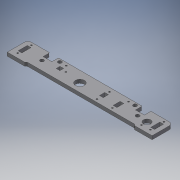
# Autodesk Inventor part: A8-0009
Saved by Autodesk Inventor 2016 SP2 (Build 200236200, 236)
## iProperties
Created: 2017-04-22
Part Number: A8-0009
Material: Generic
Document SubType Name: Modeling
Designer: EV
Density: 1 g/cm^3
Appearance: Default
Author: EV
Autodesk Inventor part; units mm, degrees
sketch "Sketch1" plane through (0, 0, 0) normal (0, 1, 0) x (-1, 0, 0)
  line L0 (-165, 47) -> (-165, 8)
  line L1 (165, 8) -> (165, 47)
  line L2 (-78, 0) -> (95.3, 0)
  line L3 (95.3, 0) -> (95.3, 15)
  line L4 (95.3, 15) -> (115.5, 15)
  line L5 (115.5, 15) -> (115.5, 0)
  line L6 (-115.5, 0) -> (-115.5, 15)
  line L7 (-115.5, 15) -> (-95.3, 15)
  line L8 (-95.3, 15) -> (-95.3, 0)
  line L9 (125, 47) -> (122, 44)
  line L10 (122, 44) -> (-122, 44)
  line L11 (-122, 44) -> (-125, 47)
  line L12 (0, 0) -> (0, 44) construction
  line L13 (165, 47) -> (125, 47)
  line L14 (-125, 47) -> (-165, 47)
  line L15 (115.5, 0) -> (157, 0)
  line L16 (-157, 0) -> (-115.5, 0)
  line L17 (-95.3, 0) -> (95.3, 0)
  line L18 (155.4, 11) -> (146.9, 11)
  line L19 (146.9, 11) -> (146.9, 32)
  line L20 (146.9, 32) -> (155.4, 32)
  line L21 (155.4, 32) -> (155.4, 11)
  line L22 (-146.9, 11) -> (-155.4, 11)
  line L23 (-155.4, 11) -> (-155.4, 32)
  line L24 (-155.4, 32) -> (-146.9, 32)
  line L25 (-146.9, 32) -> (-146.9, 11)
  line L26 (77, 15) -> (68.5, 15)
  line L27 (68.5, 15) -> (68.5, 23.5)
  line L28 (68.5, 23.5) -> (77, 23.5)
  line L29 (77, 23.5) -> (77, 15)
  line L30 (-25.6785, 15.5) -> (-34.1785, 15.5)
  line L31 (-34.1785, 15.5) -> (-34.1785, 27.5)
  line L32 (-34.1785, 27.5) -> (-25.6785, 27.5)
  line L33 (-25.6785, 27.5) -> (-25.6785, 15.5)
  line L34 (-60.7209, 15.5) -> (-69.2209, 15.5)
  line L35 (-69.2209, 15.5) -> (-69.2209, 31.5)
  line L36 (-69.2209, 31.5) -> (-60.7209, 31.5)
  line L37 (-60.7209, 31.5) -> (-60.7209, 15.5)
  arc A0 (157, 0) -> (165, 8) centre (157, 8) ccw
  arc A1 (-165, 8) -> (-157, 0) centre (-157, 8) ccw
  dimension "d0" = 330
  dimension "d1" = 47
  dimension "d2" = 45
  dimension "d3" = 3
  dimension "d4" = 40
  dimension "d5" = 49.5
  dimension "d6" = 20.2
  dimension "d8" = 15
  dimension "d9" = 11
  dimension "d10" = 9.6
  dimension "d11" = 8.5
  dimension "d12" = 21
  dimension "d13" = 8.5
  dimension "d14" = 8.5
  dimension "d15" = 8.5
  dimension "d16" = 12
  dimension "d17" = 8.5
  dimension "d18" = 16
  dimension "d19" = 95.7791
  dimension "d20" = 130.8215
  dimension "d21" = 88
  dimension "d22" = 15
  dimension "d23" = 15.5
  dimension "d24" = 15.5
  dimension "d25" = 8
  constraints: 76 end point, 24 parallel, 9 perpendicular, 8 horizontal, 7 collinear, 4 point on circle, 4 tangent, 2 centre point, 2 midpoint, 2 point on line, 1 coincident, 1 equal radius, 1 vertical, 4 other
  measures "d0" distance between parallel lines of L0 L1
  measures "d1" distance between parallel lines of L15 L13
  measures "d2" angle of L13 L9
  measures "d3" distance between parallel lines of L13 L10
  measures "d4" distance of L1.end L9.start
  measures "d5" distance between parallel lines of L1 L5
  measures "d6" distance of L3.end L4.end
  measures "d8" distance between parallel lines of L15 L4
  measures "d9" distance between parallel lines of L15 L18
  measures "d10" distance between parallel lines of L1 L21
  measures "d11" distance of L18.start L18.end
  measures "d12" distance of L20.end L18.start
  measures "d13" distance of L26.start L26.end
  measures "d14" distance of L28.end L26.start
  measures "d15" distance of L30.start L30.end
  measures "d16" distance of L32.end L30.start
  measures "d17" distance of L34.start L34.end
  measures "d18" distance of L36.end L34.start
  measures "d19" distance between parallel lines of L0 L35
  measures "d20" distance between parallel lines of L31 L0
  measures "d21" distance between parallel lines of L29 L1
  measures "d22" distance between parallel lines of L2 L26
  measures "d23" distance between parallel lines of L17 L30
  measures "d24" distance between parallel lines of L2 L34
  measures "d25" radius of A0
extrude "Extrusion1" add sketch "Sketch1" along normal blind 8
fillet "Fillet1" radius 2 8 edges at (-115.5, 4, 0) (-95.3, 4, 0) (95.3, 4, 0) (115.5, 4, 0) (-125, 4, 47) (-122, 4, 44) (122, 4, 44) (125, 4, 47)
sketch "Sketch2" plane through (0, 8, 0) normal (0, 1, 0) x (1, 0, 0)
  arc A0 (124.4142, -46.4142) -> (125.8284, -47) centre (125.8284, -45) ccw construction
  line L0 (125.8284, -47) -> (165, -47) construction
  line L1 (165, -47) -> (165, -8) construction
  arc A1 (165, -8) -> (157, 0) centre (157, -8) ccw construction
  line L2 (157, 0) -> (117.5, 0) construction
  arc A2 (117.5, 0) -> (115.5, -2) centre (117.5, -2) ccw construction
  line L3 (115.5, -2) -> (115.5, -15) construction
  line L4 (115.5, -15) -> (95.3, -15) construction
  line L5 (95.3, -15) -> (95.3, -2) construction
  arc A3 (95.3, -2) -> (93.3, 0) centre (93.3, -2) ccw construction
  line L6 (93.3, 0) -> (-93.3, 0) construction
  arc A4 (-93.3, 0) -> (-95.3, -2) centre (-93.3, -2) ccw construction
  line L7 (-95.3, -2) -> (-95.3, -15) construction
  line L8 (-95.3, -15) -> (-115.5, -15) construction
  line L9 (-115.5, -15) -> (-115.5, -2) construction
  arc A5 (-115.5, -2) -> (-117.5, 0) centre (-117.5, -2) ccw construction
  line L10 (-117.5, 0) -> (-157, 0) construction
  arc A6 (-157, 0) -> (-165, -8) centre (-157, -8) ccw construction
  line L11 (-165, -8) -> (-165, -47) construction
  line L12 (-165, -47) -> (-125.8284, -47) construction
  arc A7 (-125.8284, -47) -> (-124.4142, -46.4142) centre (-125.8284, -45) ccw construction
  line L13 (-124.4142, -46.4142) -> (-122.5858, -44.5858) construction
  arc A8 (-121.1716, -44) -> (-122.5858, -44.5858) centre (-121.1716, -46) ccw construction
  line L14 (-121.1716, -44) -> (121.1716, -44) construction
  arc A9 (122.5858, -44.5858) -> (121.1716, -44) centre (121.1716, -46) ccw construction
  line L15 (122.5858, -44.5858) -> (124.4142, -46.4142) construction
  line L16 (155.4, -11) -> (155.4, -32) construction
  line L17 (155.4, -32) -> (146.9, -32) construction
  line L18 (146.9, -32) -> (146.9, -11) construction
  line L19 (146.9, -11) -> (155.4, -11) construction
  line L20 (-146.9, -11) -> (-146.9, -32) construction
  line L21 (-146.9, -32) -> (-155.4, -32) construction
  line L22 (-155.4, -32) -> (-155.4, -11) construction
  line L23 (-155.4, -11) -> (-146.9, -11) construction
  line L24 (69.2209, -15.5) -> (69.2209, -31.5) construction
  line L25 (69.2209, -31.5) -> (60.7209, -31.5) construction
  line L26 (60.7209, -31.5) -> (60.7209, -15.5) construction
  line L27 (60.7209, -15.5) -> (69.2209, -15.5) construction
  line L28 (34.1785, -15.5) -> (34.1785, -27.5) construction
  line L29 (34.1785, -27.5) -> (25.6785, -27.5) construction
  line L30 (25.6785, -27.5) -> (25.6785, -15.5) construction
  line L31 (25.6785, -15.5) -> (34.1785, -15.5) construction
  line L32 (-68.5, -15) -> (-68.5, -23.5) construction
  line L33 (-68.5, -23.5) -> (-77, -23.5) construction
  line L34 (-77, -23.5) -> (-77, -15) construction
  line L35 (-77, -15) -> (-68.5, -15) construction
  line L36 (-165, -47) -> (-125.8284, -47) construction
  line L37 (-151.15, -47) -> (-151.15, 0) construction
  line L38 (151.15, 0) -> (151.15, -47) construction
  line L39 (29.9285, -9) -> (29.9285, -37.5) construction
  line L40 (64.9709, -15.5) -> (64.9709, -37.5) construction
  line L41 (-77, -23.5) -> (-77, -15) construction
  line L42 (-77, -19.25) -> (-59, -19.25) construction
  point P0 (0, 0)
  point P1 (-151.15, -11)
  point P2 (151.15, -11)
  point P3 (151.15, -6)
  point P4 (151.15, -37)
  point P5 (-151.15, -6)
  point P6 (-151.15, -37)
  point P7 (71, -6.5)
  point P8 (85.75, -6.5)
  point P9 (109, -24)
  point P10 (132, -38)
  point P11 (132, -25.5)
  point P12 (-85.75, -6.5)
  point P13 (-71, -6.5)
  point P14 (-109, -24)
  point P15 (29.9285, -27.5)
  point P16 (29.9285, -15.5)
  point P17 (-21.5, -25)
  dimension "d29" = 5
  dimension "d30" = 5
  dimension "d31" = 5
  dimension "d32" = 5
  dimension "d33" = 6.5
  dimension "d34" = 10
  dimension "d35" = 6
  dimension "d36" = 6.5
  dimension "d37" = 33
  dimension "d38" = 9
  dimension "d39" = 21.5
  dimension "d40" = 79.25
  dimension "d41" = 94
  dimension "d42" = 94
  dimension "d43" = 79.25
  dimension "d44" = 9.5
  dimension "d45" = 56
  dimension "d46" = 56
  dimension "d47" = 24
  dimension "d48" = 24
  dimension "d56" = 143.5
  dimension "d57" = 25
  constraints: 12 point on line, 10 end point, 6 midpoint, 3 horizontal alignment, 2 perpendicular, 1 horizontal, 1 vertical, 1 vertical alignment
  measures "d29" distance from line of L21 point (-151.15, -37)
  measures "d30" distance from line of point (-151.15, -6) L23
  measures "d31" distance from line of point (151.15, -37) L17
  measures "d32" distance from line of L19 point (151.15, -6)
  measures "d33" distance from line of L39.start L31
  measures "d34" distance from line of L29 L39.end
  measures "d35" distance from line of L25 L40.end
  measures "d36" distance from line of L6 point (71, -6.5)
  measures "d37" distance from line of point (132, -38) L1
  measures "d38" distance from line of L0 point (132, -38)
  measures "d39" distance from line of L0 point (132, -25.5)
  measures "d40" distance from line of L1 point (85.75, -6.5)
  measures "d41" distance from line of L1 point (71, -6.5)
  measures "d42" distance from line of L11 point (-71, -6.5)
  measures "d43" distance from line of L11 point (-85.75, -6.5)
  measures "d44" distance from line of L42.end L32
  measures "d45" distance from line of L1 point (109, -24)
  measures "d46" distance from line of L11 point (-109, -24)
  measures "d47" distance from line of L2 point (109, -24)
  measures "d48" distance from line of L10 point (-109, -24)
  measures "d56" distance from line of L11 point (-21.5, -25)
  measures "d57" distance from line of L6 point (-21.5, -25)
hole "Hole1" at (151.15, 8, 6) at (151.15, 8, 37) at (-151.15, 8, 6) at (-151.15, 8, 37) at (29.9285, 8, 9) at (29.9285, 8, 37.5) at (64.9709, 8, 37.5) at (71, 8, 6.5) at (132, 8, 38) at (-71, 8, 6.5) at (-59, 8, 19.25) direction (0, -1, 0) diameter 3.5 end through all
hole "Hole2" at (85.75, 8, 6.5) at (109, 8, 24) at (-85.75, 8, 6.5) at (-109, 8, 24) direction (0, -1, 0) diameter 8.5 end through all
hole "Hole3" at (-21.5, 8, 25) direction (0, -1, 0) diameter 20.5 end through all
hole "Hole4" at (132, 8, 25.5) direction (0, -1, 0) diameter 16.5 end through all
ref_plane "Work Plane1" through (-165, 8, 47) normal (0, 0, 1) x (1, 0, 0)
ref_plane "Work Plane2" through (29.9285, 8, 9) normal (-1, 0, 0) x (0, 0, 1)
ref_plane "Work Plane3" through (64.9709, 8, 15.5) normal (-1, 0, 0) x (0, 0, 1)
equation "\"d30\" = d29"
equation "\"d31\" = d29"
equation "\"d32\" = d31"
equation "\"d42\" = d41"
equation "\"d43\" = d40"
equation "\"d46\" = d45"
equation "\"d48\" = d47"
body "Solid1"
